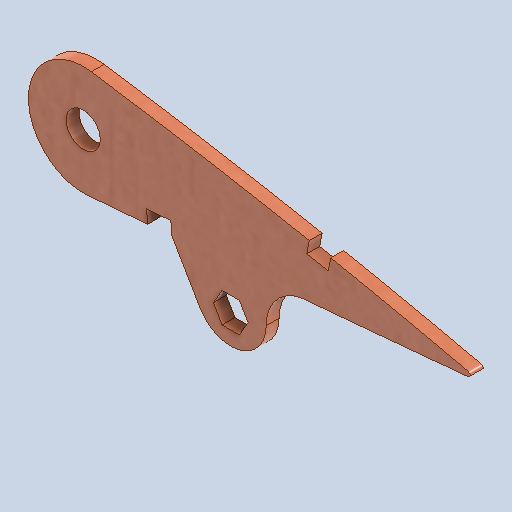
# Autodesk Inventor part: 2P.03.01.08.JW.AileronRibMid
Saved by Autodesk Inventor 2025.2 (Build 292293000, 293)
## iProperties
Created: 2024-12-05
Part Number: 2P.03.01.08.JW.AileronRibMid
Material: Wood (Walnut)
Document SubType Name: Modeling
Designer: jjrwe
Density: 0.55 g/cm^3
Appearance: Walnut - Natural Polished
Author: jjrwe
Autodesk Inventor part; units mm, degrees
ref_plane "YZ Plane" through (0, 0, 0) normal (1, 0, 0) x (0, 1, 0)
ref_plane "XZ Plane" through (0, 0, 0) normal (0, 1, 0) x (-1, 0, 0)
ref_plane "XY Plane" through (0, 0, 0) normal (0, 0, 1) x (1, 0, 0)
sketch "Sketch1" plane through (0, 0, 0) normal (0, 0, 1) x (1, 0, 0)
  spline S0 degree 2 poles (-40.9982, 18.5994) (-40.8895, 18.5833) (-40.7809, 18.5671) knots 0 0 0 1 1 1
  line L0 (-40.803, 18.5704) -> (-40.7587, 18.5638) construction
  arc A0 (-40.7631, 18.5645) -> (-40.7986, 18.5698) centre (-56.3605, -86.2568) ccw construction
  line L1 (-39.6852, 5.3344) -> (-39.4376, 2.3446)
  line L2 (-39.4376, 2.3446) -> (-33.7717, 2.8138)
  line L3 (-33.7717, 2.8138) -> (-34.0193, 5.8036)
  line L4 (-2.2691, 14.9664) -> (-1.6892, 17.9098)
  line L5 (2.7309, 13.9813) -> (-2.2691, 14.9664)
  line L6 (3.3108, 16.9248) -> (2.7309, 13.9813)
  line L7 (-1.6892, 17.9098) -> (3.3108, 16.9248)
  spline S1 degree 4 poles (-52.5686, 26.6086) (-47.4283, 25.8385) (-38.8524, 24.5329) (-27.5314, 22.6621) (-13.8317, 20.2238) (-2.8447, 18.1596) (6.9136, 16.2106) (15.3612, 14.4912) (22.3415, 12.9265) (29.1518, 11.5542) (33.1688, 10.3476) (35.6871, 10.2817) (35.9914, 9.4396) knots 0 0 0 0 0 0.183688 0.302378 0.416104 0.523956 0.624947 0.717922 0.80148 0.87369 1 1 1 1 1
  line L8 (-34.0193, 5.8036) -> (-39.6852, 5.3344)
  arc A1 (-52.5686, 26.6086) -> (-53.4266, 1.2046) centre (-54.4643, 13.9562) ccw
  circle A2 centre (-54.4643, 13.9562) radius 4
  circle A3 centre (-20.0248, -5.8183) radius 3.5
  line L9 (-33.7717, 2.8138) -> (-27.1682, -8.491)
  arc A4 (-3.3682, 5.4114) -> (-11.7521, -4.3183) centre (-1.9143, -4.3183) ccw
  arc A5 (-27.1682, -8.491) -> (-11.7521, -4.3183) centre (-20.0248, -4.3183) ccw
  spline S2 degree 4 poles (-53.4266, 1.2046) (-47.7035, 1.6704) (-39.4686, 2.3386) (-37.3837, 2.5127) (-33.7717, 2.8138) knots 0 0 0 0 0 1 1 1 1 1
  line L10 (-35.7599, 2.6481) -> (-31.7835, 2.9795) construction
  arc A6 (-32.1812, 2.9462) -> (-35.3623, 2.6811) centre (796.8879, -9962.6267) ccw construction
  spline S3 degree 4 poles (-3.3682, 5.4114) (-2.8714, 5.455) (-2.6988, 5.4696) (10.1379, 6.6067) (14.5902, 6.9981) (22.2245, 7.7443) (28.8501, 8.2309) (33.1083, 8.9133) (35.5672, 8.6498) (35.9914, 9.4396) knots 0 0 0 0 0 0.172623 0.316544 0.485874 0.63811 0.76971 1 1 1 1 1
  line L11 (-7.9773, 5.0072) -> (1.2409, 5.8157) construction
  arc A7 (0.3196, 5.7283) -> (-7.0549, 5.0815) centre (88.3466, -1040.3487) ccw construction
  line L12 (70.0994, 77.6585) -> (70.0994, -40.6368)
  line L13 (142.4679, 14.9664) -> (141.888, 17.9098)
  line L14 (137.4679, 13.9813) -> (142.4679, 14.9664)
  line L15 (136.888, 16.9248) -> (137.4679, 13.9813)
  line L16 (141.888, 17.9098) -> (136.888, 16.9248)
  spline S4 degree 4 poles (192.7674, 26.6086) (187.6271, 25.8385) (179.0512, 24.5329) (167.7302, 22.6621) (154.0305, 20.2238) (143.0435, 18.1596) (133.2852, 16.2106) (124.8376, 14.4912) (117.8573, 12.9265) (111.047, 11.5542) (107.03, 10.3476) (104.5117, 10.2817) (104.2074, 9.4396) knots 0 0 0 0 0 0.183688 0.302378 0.416104 0.523956 0.624947 0.717922 0.80148 0.87369 1 1 1 1 1
  spline S5 degree 2 poles (181.197, 18.5994) (181.0883, 18.5833) (180.9797, 18.5671) knots 0 0 0 1 1 1
  line L17 (181.0018, 18.5704) -> (180.9575, 18.5638) construction
  arc A8 (180.9974, 18.5698) -> (180.9619, 18.5645) centre (196.5593, -86.2568) ccw construction
  line L18 (173.9705, 2.8138) -> (174.2181, 5.8036)
  line L19 (174.2181, 5.8036) -> (179.8839, 5.3344)
  line L20 (179.8839, 5.3344) -> (179.6364, 2.3446)
  line L21 (179.6364, 2.3446) -> (173.9705, 2.8138)
  arc A9 (193.6254, 1.2046) -> (192.7674, 26.6086) centre (194.6631, 13.9562) ccw
  circle A10 centre (194.6631, 13.9562) radius 4
  circle A11 centre (160.2236, -5.8183) radius 3.5
  line L22 (173.9705, 2.8138) -> (167.367, -8.491)
  arc A12 (151.9509, -4.3183) -> (143.567, 5.4114) centre (142.1131, -4.3183) ccw
  arc A13 (161.3154, 3.8821) -> (160.5367, 3.9485) centre (160.2236, -4.3183) ccw
  arc A14 (151.9509, -4.3183) -> (167.367, -8.491) centre (160.2236, -4.3183) ccw
  line L23 (175.9587, 2.6481) -> (171.9823, 2.9795) construction
  arc A15 (175.5611, 2.6811) -> (172.38, 2.9462) centre (-656.6891, -9962.6267) ccw construction
  spline S6 degree 4 poles (193.6254, 1.2046) (187.9023, 1.6704) (179.6674, 2.3386) (177.5825, 2.5127) (173.9705, 2.8138) knots 0 0 0 0 0 1 1 1 1 1
  spline S7 degree 1 poles (161.3154, 3.8821) (160.5367, 3.9485) knots 0 0 1 1
  spline S8 degree 4 poles (143.567, 5.4114) (143.0702, 5.455) (142.8976, 5.4696) (130.0609, 6.6067) (125.6086, 6.9981) (117.9743, 7.7443) (111.3487, 8.2309) (107.0905, 8.9133) (104.6315, 8.6498) (104.2074, 9.4396) knots 0 0 0 0 0 0.172623 0.316544 0.485874 0.63811 0.76971 1 1 1 1 1
  line L24 (148.1761, 5.0072) -> (138.9579, 5.8157) construction
  arc A16 (147.2537, 5.0815) -> (139.8792, 5.7283) centre (51.8522, -1040.3487) ccw construction
  line L25 (-15.9834, -5.8183) -> (-18.0041, -9.3183)
  line L26 (-18.0041, -9.3183) -> (-22.0456, -9.3183)
  line L27 (-22.0456, -9.3183) -> (-24.0663, -5.8183)
  line L28 (-24.0663, -5.8183) -> (-22.0456, -2.3183)
  line L29 (-22.0456, -2.3183) -> (-18.0041, -2.3183)
  line L30 (-18.0041, -2.3183) -> (-15.9834, -5.8183)
  point P0 (0, 0)
  point P1 (-17.9436, 10.4444)
  point P2 (-26.2526, 3.4456)
  point P3 (-14.0156, 4.4896)
  point P4 (15.6814, 7.1116)
  point P5 (22.8694, 7.7686)
  point P6 (28.5454, 8.2966)
  point P7 (32.6494, 8.6836)
  point P8 (35.1304, 8.9206)
  point P9 (-38.5796, 24.4516)
  point P10 (-25.4276, 22.2616)
  point P11 (-13.2626, 20.0956)
  point P12 (-2.2076, 18.0106)
  point P13 (7.6174, 16.0606)
  point P14 (16.1074, 14.2996)
  point P15 (23.1784, 12.7756)
  point P16 (28.7524, 11.5396)
  point P17 (32.7784, 10.6276)
  point P18 (35.2084, 10.0696)
  point P19 (-67.2506, 14.3918)
  point P20 (-5.9186, 11.5242)
  point P21 (-6.911, 11.4294)
  point P22 (-8.5526, 11.2746)
  point P23 (-10.823, 11.0634)
  point P24 (-13.6982, 10.8006)
  point P25 (-17.1422, 10.4898)
  point P26 (-21.1166, 10.1382)
  point P27 (-25.577, 9.7518)
  point P28 (-30.4718, 9.3342)
  point P29 (-35.7458, 8.8938)
  point P30 (-5.8874, 11.9838)
  point P31 (-6.8594, 12.207)
  point P32 (-8.4698, 12.5718)
  point P33 (-10.6994, 13.0662)
  point P34 (-13.5278, 13.6758)
  point P35 (-16.9238, 14.3802)
  point P36 (-20.8538, 15.1602)
  point P37 (-25.2758, 15.9942)
  point P38 (-30.1418, 16.8606)
  point P39 (-35.4026, 17.7366)
  point P40 (-5.5742, 11.7318)
  point P41 (-41.3414, 8.4378)
  point P42 (35.2084, 9.4987)
  point P43 (32.7784, 9.6618)
  point P44 (28.7524, 9.9279)
  point P45 (23.1784, 10.2865)
  point P46 (16.1074, 10.7251)
  point P47 (7.6174, 11.2223)
  point P48 (-2.2076, 11.7622)
  point P49 (-13.2626, 12.3252)
  point P50 (-25.4276, 12.8888)
  point P51 (-38.5796, 13.434)
  point P52 (-52.5686, 13.9416)
  point P53 (35.9914, 8.9986)
  point P54 (-68.0606, 0.0436)
  point P55 (-67.2506, 28.6756)
  point P56 (35.9914, 9.8806)
  point P57 (140.1988, 0)
  point P58 (158.1424, 10.4444)
  point P59 (178.7784, 24.4516)
  point P60 (165.6264, 22.2616)
  point P61 (153.4614, 20.0956)
  point P62 (142.4064, 18.0106)
  point P63 (132.5814, 16.0606)
  point P64 (124.0914, 14.2996)
  point P65 (117.0204, 12.7756)
  point P66 (111.4464, 11.5396)
  point P67 (107.4204, 10.6276)
  point P68 (104.9904, 10.0696)
  point P69 (166.4514, 3.4456)
  point P70 (154.2144, 4.4896)
  point P71 (124.5174, 7.1116)
  point P72 (117.3294, 7.7686)
  point P73 (111.6534, 8.2966)
  point P74 (107.5494, 8.6836)
  point P75 (105.0684, 8.9206)
  point P76 (207.4494, 14.3918)
  point P77 (104.2074, 9.8806)
  point P78 (207.4494, 28.6756)
  point P79 (208.2594, 0.0436)
  point P80 (104.2074, 8.9986)
  point P81 (192.7674, 13.9416)
  point P82 (178.7784, 13.434)
  point P83 (165.6264, 12.8888)
  point P84 (153.4614, 12.3252)
  point P85 (142.4064, 11.7622)
  point P86 (132.5814, 11.2223)
  point P87 (124.0914, 10.7251)
  point P88 (117.0204, 10.2865)
  point P89 (111.4464, 9.9279)
  point P90 (107.4204, 9.6618)
  point P91 (104.9904, 9.4987)
  point P92 (181.5402, 8.4378)
  point P93 (145.773, 11.7318)
  point P94 (175.6014, 17.7366)
  point P95 (170.3406, 16.8606)
  point P96 (165.4746, 15.9942)
  point P97 (161.0526, 15.1602)
  point P98 (157.1226, 14.3802)
  point P99 (153.7266, 13.6758)
  point P100 (150.8982, 13.0662)
  point P101 (148.6686, 12.5718)
  point P102 (147.0582, 12.207)
  point P103 (146.0862, 11.9838)
  point P104 (175.9446, 8.8938)
  point P105 (170.6706, 9.3342)
  point P106 (165.7758, 9.7518)
  point P107 (161.3154, 10.1382)
  point P108 (157.341, 10.4898)
  point P109 (153.897, 10.8006)
  point P110 (151.0218, 11.0634)
  point P111 (148.7514, 11.2746)
  point P112 (147.1098, 11.4294)
  point P113 (146.1174, 11.5242)
  dimension "d0" = 3
  dimension "d1" = 5
  dimension "d2" = 52.7751
  dimension "d3" = 3
  dimension "d4" = 5.6658
  dimension "d9" = 8
  dimension "d11" = 7
  constraints: 95 symmetric about line, 62 end point, 22 point on circle, 17 centre point, 9 midpoint, 4 parallel, 3 coincident, 2 perpendicular, 2 point on line, 2 tangent, 1 vertical, 93 other
  measures "d0" distance of L6.start L5.start
  measures "d1" horizontal distance of L6.start L4.end
  measures "d2" horizontal distance of A1.centre L4.end
  measures "d3" distance of L3.end L3.start
  measures "d4" horizontal distance of L3.end L8.end
  measures "d9" diameter of A2
  measures "d11" diameter of A3
extrude "Extrusion2" add sketch "Sketch1" along normal blind 3 contours L1 S2 A1 S1 L4 L5 L6 S3 A4 A5 L9 L3 L8
body "Solid2"
